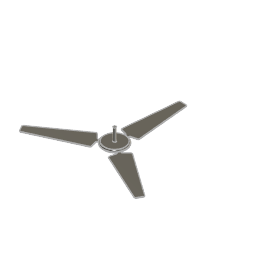
Ceiling Fan (Autodesk Fusion 360 design; units mm, degrees)
part number: 2026-03-22-21-24-57-031
part number: 2026-03-22-21-37-14-324
part number: 2026-03-22-21-38-04-860
part number: 2026-03-22-21-56-55-715
Autodesk Fusion 360 part; units mm, degrees
sketch "Sketch1" plane through (0, 0, 0) normal (0, 0, 1) x (1, 0, 0)
  circle A0 centre (0, 0) radius 75
  line L0 (0, 75) -> (0, -75) construction
  line L1 (0, 0) -> (-37.5, -64.9519) construction
  line L2 (0, 0) -> (37.5, -64.9519) construction
  dimension "d1" = 150
  dimension "d3" = 60
  constraint coincident A0.centre L1.start
  constraint coincident A0 L0.start
  constraint coincident A0 L0.end
  constraint vertical L0
  constraint coincident A0 L1.end
  constraint coincident A0 L2.end
  measures "d1" diameter of A0
  measures "d3" angle of L1 L2
extrude "Extrude1" add sketch "Sketch1" against normal blind 20 makes body 1
ref_plane "WorkPlane1" through (0, 75, 0) normal (0, 1, 0) x (0, 0, 1)
sketch "Sketch4" plane through (0, 75, 0) normal (0, 1, 0) x (1, 0, 0)
  line L0 (12.5, 10) -> (-12.5, 10)
  line L1 (-12.5, 10) -> (-12.5, 14)
  line L2 (-12.5, 14) -> (12.5, 14)
  line L3 (12.5, 14) -> (12.5, 10)
  line L4 (75, 20) -> (-75, 20)
  line L5 (-75, 0) -> (75, 0)
  line L6 (-75, 0) -> (75, 0)
  point P0 (0, 10)
  dimension "d7" = 25
  dimension "d8" = 4
  dimension "d9" = 10
  constraint horizontal L0
  constraint vertical L1
  constraint horizontal L2
  constraint vertical L3
  constraint midpoint L0 P0
  constraint vertical P0 origin
  measures "d7" distance of L1 L3
  measures "d8" distance of L0.end L1.end
  measures "d9" distance of L0 L6
extrude "Extrude2" cut sketch "Sketch4" against normal blind 25 bodies 1
pattern_circular "C-Pattern1" count 3 over 360 about axis through (0, 0, 1.75) along (0, 0, 1) of "Extrude2"
copy_body "Body->Comp1" bodies 1 removing the originals makes body 2 in component "Circular ring"
sketch "Sketch1 (2)" plane through (0, 0, 0) normal (0, 0, 1) x (1, 0, 0) in component "blade"
  line L0 (0.8744, -6.3253) -> (0.8744, 28.6747)
  line L1 (0.8744, 28.6747) -> (49.0748, 41.9683)
  line L2 (49.0748, 41.9683) -> (15.8744, 391.9683)
  line L3 (15.8744, 391.9683) -> (-34.1256, 391.9683)
  line L4 (-34.1256, 391.9683) -> (-67.3261, 41.9683)
  line L5 (-67.3261, 41.9683) -> (-19.1256, 28.6747)
  line L6 (-19.1256, 28.6747) -> (-19.1256, -6.3253)
  line L7 (-19.1256, -6.3253) -> (0.8744, -6.3253)
  point P0 (-9.1256, -6.3253)
  point P1 (-9.1256, 391.9683)
  dimension "d14" = 350
  dimension "d15" = 20
  dimension "d16" = 50
  dimension "d17" = 50
  dimension "d34" = 35
  dimension "d35" = 100
  constraint vertical L0
  constraint perpendicular L0 L3
  constraint parallel L0 L6
  constraint perpendicular L0 L7
  constraint equal L1 L5
  constraint equal L0 L6
  constraint equal L2 L4
  constraint midpoint L7 P0
  constraint midpoint L3 P1
  constraint vertical P0 P1
  measures "d14" vertical distance of L3.end L4.end
  measures "d15" distance of L0.start L6.end
  measures "d16" distance of L0.end L1.end
  measures "d17" distance of L2.end L3.end
  measures "d34" distance of L5.end L6.end
  measures "d35" angle of L4 L5
fillet "Fillet1" radius 8 2 faces at (17.4948, 13.3615, 0) (17.4948, 13.3615, -20) on bodies 2 in component "Circular ring"
extrude "Extrude2'" add sketch "Sketch1 (2)" against normal blind 4 separate body makes body 3 in component "blade"
fillet "Fillet3" radius 6 6 edges at (0.8744, -6.3253, -2) (-19.1256, 28.6747, -2) (0.8744, 28.6747, -2) (49.0748, 41.9683, -2) (-67.3261, 41.9683, -2) (-19.1256, -6.3253, -2) on bodies 3 in component "blade"
fillet "Fillet3" radius 8 2 edges at (15.8744, 391.9683, -2) (-34.1256, 391.9683, -2) on bodies 3 in component "blade"
fillet "Fillet4" radius 0.125 32 edges at (13.9804, 389.8863, 0) (-9.1256, 391.9683, 0) (-32.2317, 389.8863, 0) (-50.8317, 215.8521, 0) (-65.8174, 43.0084, 0) (-43.0015, 35.2597, 0) (-20.3522, 27.7407, 0) (-19.1256, 11.8901, 0) (-17.3683, -4.5679, 0) (-9.1256, -6.3253, 0) (-0.883, -4.5679, 0) (0.8744, 11.8901, 0) (2.1009, 27.7407, 0) (24.7503, 35.2597, 0) (47.5661, 43.0084, 0) (32.5805, 215.8521, 0) (47.5661, 43.0084, -4) (24.7503, 35.2597, -4) (2.1009, 27.7407, -4) (0.8744, 11.8901, -4) (-0.883, -4.5679, -4) (-9.1256, -6.3253, -4) (-17.3683, -4.5679, -4) (-19.1256, 11.8901, -4) (-20.3522, 27.7407, -4) (-43.0015, 35.2597, -4) (-65.8174, 43.0084, -4) (-50.8317, 215.8521, -4) (-32.2317, 389.8863, -4) (-9.1256, 391.9683, -4) (13.9804, 389.8863, -4) (32.5805, 215.8521, -4) on bodies 3 in component "blade"
sketch "Sketch5" plane through (-9.1256, -56.3253, 10) normal (0, 0, 1) x (0.5, -0.866025, 0)
  circle A0 centre (0, 0) radius 67
  circle A1 centre (0, 0) radius 10
  dimension "d48" = 20
  constraint concentric A0 A1
  measures "d48" diameter of A1
sketch "Sketch1 (3)" plane through (-9.1256, -56.3253, 10) normal (0, 0, 1) x (0.5, -0.866025, 0) in component "ConRod"
  circle A0 centre (0, 0) radius 67
  circle A1 centre (0, 0) radius 9.25
  dimension "d51" = 18.5
  constraint concentric A0 A1
  measures "d51" diameter of A1
extrude "Extrude1'" add sketch "Sketch1 (3)" along normal blind 80 separate body contours A1 makes body 4 in component "ConRod"
component "blade" placed x (-0.5, -0.866025, 0) y (-0.866025, 0.5, 0) z (0, 0, -1) at (-62.4676, -36.0657, 100)
component "Circular ring" placed x (1, 0, 0) y (0, -1, 0) z (0, 0, -1) at (-9.1256, -56.3253, 90)
component "blade" placed x (1, 0, 0) y (0, -1, 0) z (0, 0, -1) at (0, -112.6505, 100)
component "blade" placed x (-0.5, 0.866025, 0) y (0.866025, 0.5, 0) z (0, 0, -1) at (35.0907, -20.2596, 100)
component "ConRod" placed x (1, 0, 0) y (0, 1, 0) z (0, 0, 1) at (0, 0, 0)
